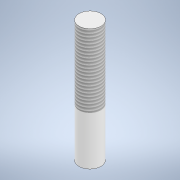
# Autodesk Inventor part: shaftucu2
Saved by Autodesk Inventor 2020 (Build 240168000, 168)
## iProperties
Created: 2021-12-07
Part Number: shaftucu2
Material: ABS Plastic
Document SubType Name: Modeling
Designer: Umur Batuhan Özmen
Density: 1.06 g/cm^3
Appearance: Smooth - White
Mass: 3.37171 g
Surface Area: 15.4095 cm^2
Volume: 3.18086 cm^3
Author: Umur Batuhan Özmen
## iProperties of the stored document _3DPrint.ipt
Created: 2021-12-10
Part Number: _3DPrint
Material: Generic
Document SubType Name: Modeling
Designer: Umur Batuhan Özmen
Density: 1 g/cm^3
Appearance: Default
Author: Umur Batuhan Özmen
Autodesk Inventor part; units mm, degrees
ref_plane "YZ Plane" through (0, 0, 0) normal (1, 0, 0) x (0, 1, 0)
ref_plane "XZ Plane" through (0, 0, 0) normal (0, 1, 0) x (-1, 0, 0)
ref_plane "XY Plane" through (0, 0, 0) normal (0, 0, 1) x (1, 0, 0)
sketch "Sketch1" plane through (0, 0, 0) normal (0, 1, 0) x (-1, 0, 0)
  circle A0 centre (0, 0) radius 4.5
  dimension "d0" = 9
  constraints: 1 centre point, 1 coincident
  measures "d0" diameter of A0
extrude "Extrusion1" add sketch "Sketch1" along normal blind 30
sketch "Sketch3" plane through (0, 30, 0) normal (0, 1, 0) x (1, 0, 0)
  circle A0 centre (0, 0) radius 4.5 projected
  circle A1 centre (0, 0) radius 4.4
  constraints: 1 centre point, 1 coincident
extrude "Extrusion2" add sketch "Sketch3" along normal blind 20 contours A0 | A1
thread "Thread2" size "M9x1.25" class "6g" standard "ANSI Metric M Profile" length 30
body "Solid1"
